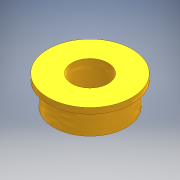
# Autodesk Inventor part: ベアリング　内径5 外径10
Saved by Autodesk Inventor 2020.2 (Build 242310000, 310)
## iProperties
Created: 2018-03-28
Part Number: ベアリング　内径5 外径10
Material: 一般
Document SubType Name: Modeling
Designer: Takumi
Mass: 1.46 g
Surface Area: 3.64613 cm^2
Volume: 0.257334 cm^3
Density: 5.67356 g/cm^3
Appearance: 溶接 - 真鍮
Author: Takumi
Autodesk Inventor part; units mm, degrees
ref_plane "YZ Plane" through (0, 0, 0) normal (1, 0, 0) x (0, 1, 0)
ref_plane "XZ Plane" through (0, 0, 0) normal (0, 1, 0) x (-1, 0, 0)
ref_plane "XY Plane" through (0, 0, 0) normal (0, 0, 1) x (1, 0, 0)
sketch "スケッチ1" plane through (0, 0, 0) normal (0, 0, 1) x (1, 0, 0)
  circle A0 centre (0, 0) radius 2.5
  circle A1 centre (0, 0) radius 5
  circle A2 centre (0, 0) radius 5.8
  dimension "d0" = 5
  dimension "d1" = 10
  dimension "d2" = 11.6
  constraints: 3 centre point, 3 coincident
  measures "d0" diameter of A0
  measures "d1" diameter of A1
  measures "d2" diameter of A2
extrude "押し出し1" add sketch "スケッチ1" along normal blind 0.8 contours A1 | A2
extrude "押し出し2" add sketch "スケッチ1" against normal blind 3.2 contours A1
